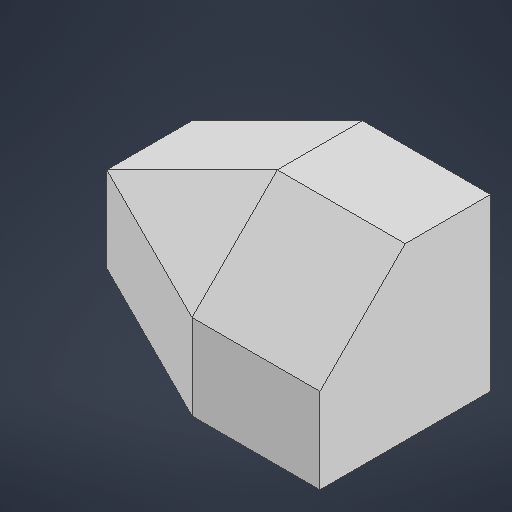
# Autodesk Inventor part: B7
Saved by Autodesk Inventor 2025.4 (Build 294407000, 407)
## iProperties
Created: 2026-05-14
Part Number: B7
Material: Generic
Document SubType Name: Modeling
Designer: VuQuan
Density: 1 g/cm^3
Appearance: Default
Author: VuQuan
Autodesk Inventor part; units mm, degrees
ref_plane "YZ Plane" through (0, 0, 0) normal (1, 0, 0) x (0, 1, 0)
ref_plane "XZ Plane" through (0, 0, 0) normal (0, 1, 0) x (-1, 0, 0)
ref_plane "XY Plane" through (0, 0, 0) normal (0, 0, 1) x (1, 0, 0)
sketch "Sketch1" plane through (0, 0, 0) normal (0, 0, 1) x (1, 0, 0)
  line L0 (0, 0) -> (0, 20)
  line L1 (0, 20) -> (40, 40)
  line L2 (40, 40) -> (70, 40)
  line L3 (70, 40) -> (70, 0)
  line L4 (70, 0) -> (0, 0)
  dimension "d0" = 70
  dimension "d1" = 40
  dimension "d2" = 20
  dimension "d3" = 30
  constraints: 10 end point, 3 perpendicular, 1 vertical
  measures "d0" distance between parallel lines of L3 L0
  measures "d1" distance of L2.end L3.end
  measures "d2" distance of L0.start L0.end
  measures "d3" distance of L1.end L2.end
extrude "Extrusion1" add sketch "Sketch1" along normal blind 40
sketch "Sketch2" plane through (0, 0, 0) normal (0, -1, 0) x (1, 0, 0)
  line L0 (0, 40) -> (70, 40) projected
  line L1 (0, 0) -> (0, 40) projected
  line L2 (0, 0) -> (0, 40) projected
  line L3 (0, 20) -> (40, 40)
  constraints: 2 end point, 1 midpoint
extrude "Extrusion2" cut sketch "Sketch2" against normal through all
sketch "Sketch3" plane through (70, 0, 0) normal (1, 0, 0) x (0, 0, -1)
  line L0 (0, 40) -> (-40, 40) projected
  line L1 (-40, 0) -> (-40, 40) projected
  line L2 (-20, 40) -> (-40, 20)
  constraints: 2 end point, 2 midpoint
extrude "Extrusion3" cut sketch "Sketch3" against normal through all
sketch "Sketch4" plane through (40, 20, 40) normal (0, 0.7071, 0.7071) x (1, 0, 0)
  line L0 (-20, 14.1421) -> (0, 28.2843) projected
  line L1 (0, 0) -> (-20, 14.1421) projected
  line L2 (0, 28.2843) -> (0, 0)
  point P0 (-40, 14.1421)
  constraints: 2 end point, 1 vertical
sketch "Sketch5" plane through (0, 20, 20) normal (-0.4472, 0.8944, 0) x (0.8944, 0.4472, 0)
  line L0 (-8.9443, 0) -> (0, 0) projected
  line L1 (44.7214, 0) -> (0, 0)
  point P0 (-8.9443, 20)
  constraints: 2 end point, 1 collinear
sweep "Sweep1" cut profiles "Sketch4" path "Sketch5" path curves L1
body "Solid1"
